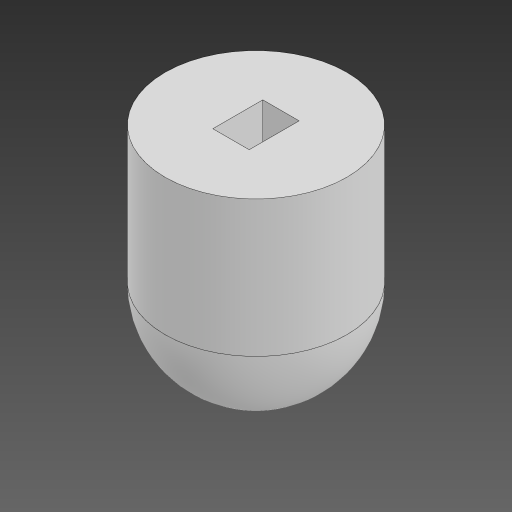
# Autodesk Inventor part: Joy
Saved by Autodesk Inventor 2023.2 (Build 272271000, 271)
## iProperties
Created: 2023-06-12
Part Number: Joy
Material: Generic
Document SubType Name: Modeling
Designer: jcgg2
Mass: 0.418034 g
Surface Area: 3.39593 cm^2
Volume: 0.418034 cm^3
Density: 1 g/cm^3
Appearance: Default
Author: jcgg2
Autodesk Inventor part; units mm, degrees
ref_plane "YZ Plane" through (0, 0, 0) normal (1, 0, 0) x (0, 1, 0)
ref_plane "XZ Plane" through (0, 0, 0) normal (0, 1, 0) x (-1, 0, 0)
ref_plane "XY Plane" through (0, 0, 0) normal (0, 0, 1) x (1, 0, 0)
sketch "Sketch1" plane through (0, 0, 0) normal (0, 1, 0) x (-1, 0, 0)
  line L0 (-0.8, 1.1) -> (0.8, 1.1)
  line L1 (0.8, 1.1) -> (0.8, -1.1)
  line L2 (0.8, -1.1) -> (-0.8, -1.1)
  line L3 (-0.8, -1.1) -> (-0.8, 1.1)
  line L4 (-0.8, 1.1) -> (0.8, -1.1) construction
  line L5 (0.8, 1.1) -> (-0.8, -1.1) construction
  circle A0 centre (0, 0) radius 4
  dimension "d0" = 1.6
  dimension "d1" = 2.2
  dimension "d2" = 8
  constraints: 12 end point, 2 midpoint, 2 parallel, 1 centre point, 1 coincident, 1 horizontal, 1 perpendicular
  measures "d0" distance of L1.end L2.end
  measures "d1" distance of L0.end L1.end
  measures "d2" diameter of A0
extrude "Extrusion1" add sketch "Sketch1" along normal blind 10
extrude "Extrusion2" add sketch "Sketch1" along normal blind 5 contours L0 L1 L2 L3
fillet "Fillet1" radius 4 1 edges at (4, 0, 0)
body "Solid1"
